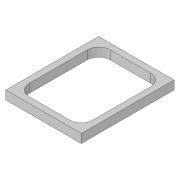
# Autodesk Inventor part: cellSTORM_chip_chamber
Saved by Autodesk Inventor 2019.4 (Build 234330000, 330)
## iProperties
Created: 2020-06-30
Part Number: cellSTORM_chip_chamber
Material: Generic
Document SubType Name: Modeling
Designer: diederichbenedict
Density: 1 g/cm^3
Appearance: Default
Author: diederichbenedict
Autodesk Inventor part; units mm, degrees
ref_plane "YZ Plane" through (0, 0, 0) normal (1, 0, 0) x (0, 1, 0)
ref_plane "XZ Plane" through (0, 0, 0) normal (0, 1, 0) x (-1, 0, 0)
ref_plane "XY Plane" through (0, 0, 0) normal (0, 0, 1) x (1, 0, 0)
sketch "Sketch1" plane through (0, 0, 0) normal (0, 1, 0) x (-1, 0, 0)
  line L0 (6.5, -8) -> (-6.5, -8)
  line L1 (-6.5, -8) -> (-6.5, 8)
  line L2 (-6.5, 8) -> (6.5, 8)
  line L3 (6.5, 8) -> (6.5, -8)
  line L4 (6.5, -8) -> (-6.5, 8) construction
  line L5 (-6.5, -8) -> (6.5, 8) construction
  line L6 (5.5, -7) -> (-5.5, -7)
  line L7 (-5.5, -7) -> (-5.5, 7)
  line L8 (-5.5, 7) -> (5.5, 7)
  line L9 (5.5, 7) -> (5.5, -7)
  point P0 (0, 0)
  dimension "d0" = 13
  dimension "d1" = 16
  dimension "d2" = 1
  constraints: 20 end point, 4 parallel, 2 midpoint, 2 perpendicular, 1 horizontal, 3 other
  measures "d0" distance of L1.end L2.end
  measures "d1" distance of L0.end L1.end
  measures "d2" distance between parallel lines of L3 L9
extrude "Extrusion1" add sketch "Sketch1" along normal blind 1.5
fillet "Fillet1" radius 2 4 edges at (-5.5, 0.75, -7) (-5.5, 0.75, 7) (5.5, 0.75, 7) (5.5, 0.75, -7)
body "Solid1"
